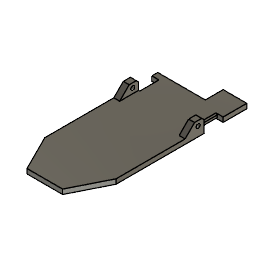
Ball Flick Thing (Autodesk Fusion 360 design; units mm, degrees)
Autodesk Fusion 360 part; units mm, degrees
sketch "Sketch1" plane through (0, 0, 0) normal (0, 0, 1) x (1, 0, 0)
  line L0 (30, -70) -> (-30, -70)
  line L1 (-30, -70) -> (-30, 70)
  line L2 (-30, 70) -> (30, 70)
  line L3 (30, 70) -> (30, -70)
  line L4 (30, -70) -> (-30, 70) construction
  line L5 (-30, -70) -> (30, 70) construction
  line L6 (-30, 70) -> (10, 70)
  line L7 (10, 70) -> (10, 55)
  line L8 (10, 55) -> (-30, 55)
  line L9 (-30, 55) -> (-30, 70)
  line L10 (-30, 50) -> (-25, 50)
  line L11 (-25, 50) -> (-25, 34)
  line L12 (-25, 34) -> (-30, 34)
  line L13 (-30, 34) -> (-30, 50)
  line L14 (0, 1.75) -> (0, 22.5)
  line L15 (30, 50) -> (25, 50)
  line L16 (25, 50) -> (25, 34)
  line L17 (25, 34) -> (30, 34)
  line L18 (-30, 34) -> (-25, 34)
  line L19 (-25, 34) -> (-25, 24)
  line L20 (-25, 24) -> (-30, 24)
  line L21 (-30, 24) -> (-30, 34)
  line L22 (25, 34) -> (25, 24)
  line L23 (25, 24) -> (30, 24)
  line L24 (25, 34) -> (30, 34)
  dimension "d1" = 60
  dimension "d2" = 140
  dimension "d3" = 40
  dimension "d4" = 15
  dimension "d5" = 5
  dimension "d6" = 16
  dimension "d7" = 5
  dimension "d8" = 5
  dimension "d9" = 10
  constraint horizontal L0
  constraint perpendicular L0 L1
  constraint parallel L0 L2
  constraint parallel L1 L3
  constraint coincident L4 origin
  constraint coincident L5 origin
  constraint horizontal L6
  constraint vertical L7
  constraint horizontal L8
  constraint vertical L9
  constraint horizontal L10
  constraint vertical L11
  constraint horizontal L12
  constraint vertical L13
  constraint coincident L1 L10.start
  constraint symmetric L10.start L14 L15.start
  constraint symmetric L10.end L14 L15.end
  constraint symmetric L11.end L14 L16.end
  constraint symmetric L12.end L14 L17.end
  constraint horizontal L18
  constraint vertical L19
  constraint horizontal L20
  constraint vertical L21
  constraint symmetric L14 L11.end L16.end
  constraint symmetric L14 L19.end L22.end
  constraint symmetric L14 L20.end L23.end
  measures "d1" distance of L1.end L2.end
  measures "d2" distance of L0.end L1.end
  measures "d3" distance of L1.end L6.end
  measures "d4" distance of L1.end L8.end
  measures "d5" distance of L10.start L10.end
  measures "d6" distance of L10.start L12.end
  measures "d7" distance of L8 L10
  measures "d8" distance of L12.end L11.end
  measures "d9" distance of L12.end L20.end
extrude "Extrude1" add sketch "Sketch1" along normal blind 4 contours L0 L1 L2 L3 L7 L8 L10 L11 L15 L16 L19 L20 L22 L23
extrude "Extrude2" add sketch "Sketch1" along normal blind 12 contours L3 L17 L22 L23 L24 | L1 L12 L18 L19 L20 L21
chamfer "Chamfer1" distance 15 distance2 30 1 edges at (30, -70, 2) measured on face at (10, -70, 1.3333)
chamfer "Chamfer1" distance 30 distance2 15 1 edges at (-30, -70, 2) measured on face at (-30, 30.6667, 5.3333)
chamfer "Chamfer1" distance 1 distance2 1 4 edges at (-25, 42, 0) (-25, 42, 4) (25, 42, 4) (25, 42, 0) measured on face at (-25, 44.6667, 1.3333) measured on face at (-8.3333, -38.6667, 4) measured on face at (-8.3333, -38.6667, 4) measured on face at (-8.3333, -35.3333, 0)
chamfer "Chamfer1" distance 6 distance2 6 2 edges at (27.5, 24, 4) (-27.5, 24, 4) measured on face at (-8.3333, -38.6667, 4) measured on face at (-8.3333, -38.6667, 4)
chamfer "Chamfer1" distance 2 distance2 2 4 edges at (27.5, 24, 12) (27.5, 34, 12) (-27.5, 24, 12) (-27.5, 34, 12) measured on face at (28.3333, 30.6667, 12) measured on face at (28.3333, 30.6667, 12) measured on face at (-28.3333, 30.6667, 12) measured on face at (-28.3333, 30.6667, 12)
sketch "Sketch2" plane through (0, 0, 0) normal (1, 0, 0) x (0, 1, 0)
  circle A0 centre (29, 8) radius 1.7
  dimension "d22" = 3.4
  dimension "d23" = 29
  dimension "d24" = 8
  measures "d22" diameter of A0
  measures "d23" horizontal distance of origin A0.centre
  measures "d24" vertical distance of origin A0.centre
extrude "Extrude3" cut sketch "Sketch2" along normal mid plane 100
